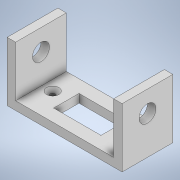
# Autodesk Inventor part: 1st arm to 2nd linking clamp
Saved by Autodesk Inventor 2022 (Build 260153000, 153)
## iProperties
Created: 2021-06-29
Part Number: 1st arm to 2nd linking clamp
Material: Generic
Document SubType Name: Modeling
Designer: USER
Density: 1 g/cm^3
Appearance: Default
Author: USER
Autodesk Inventor part; units mm, degrees
ref_plane "YZ Plane" through (0, 0, 0) normal (1, 0, 0) x (0, 1, 0)
ref_plane "XZ Plane" through (0, 0, 0) normal (0, 1, 0) x (-1, 0, 0)
ref_plane "XY Plane" through (0, 0, 0) normal (0, 0, 1) x (1, 0, 0)
sketch "Sketch1" plane through (0, 0, 0) normal (0, 0, 1) x (1, 0, 0)
  line L0 (0, 0) -> (0, 35)
  line L1 (0, 35) -> (5, 35)
  line L2 (5, 35) -> (5, 5)
  line L3 (5, 5) -> (63, 5)
  line L4 (63, 5) -> (63, 35)
  line L5 (63, 35) -> (68, 35)
  line L6 (68, 35) -> (68, 0)
  line L7 (68, 0) -> (0, 0)
  dimension "d0" = 35
  dimension "d1" = 5
  dimension "d2" = 30
  dimension "d3" = 58
  dimension "d4" = 30
  dimension "d5" = 5
  constraints: 16 end point, 6 perpendicular, 2 vertical
  measures "d0" distance of L0.start L0.end
  measures "d1" distance of L0.end L1.end
  measures "d2" distance of L1.end L2.end
  measures "d3" distance of L2.end L3.end
  measures "d4" distance of L3.end L4.end
  measures "d5" distance of L4.end L5.end
extrude "Extrusion1" add sketch "Sketch1" along normal blind 30
sketch "Sketch2" plane through (68, 0, 0) normal (1, 0, 0) x (0, 0, -1)
  circle A0 centre (-15, 22.5) radius 5
  line L0 (0, 35) -> (-30, 35) projected
  line L1 (0, 0) -> (0, 35) projected
  dimension "d8" = 10
  dimension "d9" = 12.5
  dimension "d10" = 15
  constraints: 1 centre point
  measures "d8" diameter of A0
  measures "d9" distance from line of L0 A0.centre
  measures "d10" distance from line of L1 A0.centre
extrude "Extrusion2" cut sketch "Sketch2" against normal through all
sketch "Sketch3" plane through (5, 5, 0) normal (0, 1, 0) x (1, 0, 0)
  line L0 (15, -22.5) -> (43, -22.5)
  line L1 (43, -22.5) -> (43, -7.5)
  line L2 (43, -7.5) -> (15, -7.5)
  line L3 (15, -7.5) -> (15, -22.5)
  line L4 (15, -22.5) -> (43, -7.5) construction
  line L5 (43, -22.5) -> (15, -7.5) construction
  line L6 (58, 0) -> (0, 0) projected
  line L7 (0, 0) -> (0, -30) projected
  point P0 (-5, 0)
  point P1 (29, -15)
  dimension "d13" = 28
  dimension "d14" = 15
  dimension "d15" = 15
  dimension "d16" = 29
  constraints: 12 end point, 2 midpoint, 2 parallel, 1 horizontal, 1 perpendicular
  measures "d13" distance of L2.end L1.end
  measures "d14" distance of L1.end L0.end
  measures "d15" distance from line of L6 point (29, -15)
  measures "d16" distance from line of L7 point (29, -15)
extrude "Extrusion3" cut sketch "Sketch3" against normal through all
sketch "Sketch4" plane through (5, 5, 0) normal (0, 1, 0) x (1, 0, 0)
  circle A0 centre (6, -14.0611) radius 3.625
  line L0 (0, -10) -> (0, -20) projected
  circle A1 centre (52, -14.0611) radius 3.625
  line L1 (43, -7.5) -> (43, -22.5) projected
  point P0 (-5, 0)
  dimension "d19" = 7.25
  dimension "d20" = 6
  dimension "d21" = 7.25
  dimension "d22" = 9
  constraints: 2 centre point
  measures "d19" diameter of A0
  measures "d20" distance from line of L0 A0.centre
  measures "d21" diameter of A1
  measures "d22" distance from line of L1 A1.centre
extrude "Extrusion4" cut sketch "Sketch4" against normal blind 2.1735 draft -45
sketch "Sketch5" plane through (11, 2.8265, 14.0611) normal (0, 1, 0) x (1, 0, 0)
  circle A0 centre (0, 0) radius 1.4515
  circle A1 centre (46, 0) radius 1.4515 projected
  circle A2 centre (46, 0) radius 1.4515
  point P0 (-11, 14.0611)
  constraints: 2 centre point, 1 coincident
extrude "Extrusion5" cut sketch "Sketch5" against normal through all
sketch "Sketch6" plane through (5, 5, 0) normal (0, 1, 0) x (1, 0, 0)
  point P0 (-5, 0)
body "Solid1"
